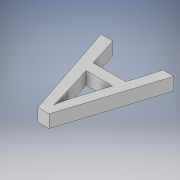
# Autodesk Inventor part: Letter_A
Saved by Autodesk Inventor 2019 (Build 230136000, 136)
## iProperties
Created: 2019-03-06
Part Number: Letter_A
Material: Generic
Document SubType Name: Modeling
Designer: jmc
Density: 1 g/cm^3
Appearance: Default
Author: jmc
## iProperties of the stored document Letter_A_3DPrint.ipt
Created: 2019-03-06
Part Number: Letter_A_3DPrint
Material: Generic
Document SubType Name: Modeling
Designer: jmc
Density: 1 g/cm^3
Appearance: Default
Author: jmc
Autodesk Inventor part; units mm, degrees
ref_plane "YZ Plane" through (0, 0, 0) normal (1, 0, 0) x (0, 1, 0)
ref_plane "XZ Plane" through (0, 0, 0) normal (0, 1, 0) x (-1, 0, 0)
ref_plane "XY Plane" through (0, 0, 0) normal (0, 0, 1) x (1, 0, 0)
sketch "Sketch1" plane through (0, 0, 0) normal (0, 1, 0) x (-1, 0, 0)
  line L0 (7.8064, 7.8064) -> (173.9884, 7.8064) construction
  line L1 (173.9884, 7.8064) -> (173.9884, -141.9122) construction
  line L2 (173.9884, -141.9122) -> (7.8064, -141.9122) construction
  line L3 (7.8064, -141.9122) -> (7.8064, 7.8064) construction
  line L4 (7.5748, -142.1936) -> (54.8334, 7.8064)
  line L5 (54.8334, 7.8064) -> (72.4396, 7.8064)
  line L6 (72.4396, 7.8064) -> (122.7099, -142.1936)
  line L7 (122.7099, -142.1936) -> (104.0612, -142.1936)
  line L8 (104.0612, -142.1936) -> (89.8141, -96.7882)
  line L9 (89.8141, -96.7882) -> (38.1539, -96.7882)
  line L10 (38.1539, -96.7882) -> (24.8334, -142.1936)
  line L11 (24.8334, -142.1936) -> (7.5748, -142.1936)
  line L12 (42.9029, -80.572) -> (84.7176, -80.572)
  line L13 (84.7176, -80.572) -> (71.9763, -38.989)
  spline S0 degree 2 poles (71.9763, -38.989) (65.9531, -19.877) (63.289, -7.9465) knots 0 0 0 1 1 1
  spline S1 degree 2 poles (63.289, -7.9465) (60.8566, -22.4252) (56.5709, -36.5565) knots 0 0 0 1 1 1
  line L14 (56.5709, -36.5565) -> (42.9029, -80.572)
  point P0 (0, 0)
  constraints: 2 other
extrude "Extrusion1" add sketch "Sketch1" along normal blind 20
body "Solid1"
